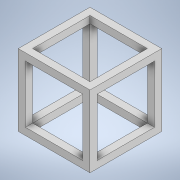
# Autodesk Inventor part: Hollow_Cube
Saved by Autodesk Inventor 2020 (Build 240168000, 168)
## iProperties
Created: 2021-12-24
Part Number: Hollow_Cube
Material: Generic
Document SubType Name: Modeling
Designer: Umur Batuhan Özmen
Density: 1 g/cm^3
Appearance: Default
Author: Umur Batuhan Özmen
Autodesk Inventor part; units mm, degrees
ref_plane "YZ Plane" through (0, 0, 0) normal (1, 0, 0) x (0, 1, 0)
ref_plane "XZ Plane" through (0, 0, 0) normal (0, 1, 0) x (-1, 0, 0)
ref_plane "XY Plane" through (0, 0, 0) normal (0, 0, 1) x (1, 0, 0)
sketch "Sketch1" plane through (0, 0, 0) normal (0, 1, 0) x (-1, 0, 0)
  line L0 (50, 50) -> (-50, 50)
  line L1 (-50, 50) -> (-50, -50)
  line L2 (-50, -50) -> (50, -50)
  line L3 (50, -50) -> (50, 50)
  line L4 (50, 50) -> (-50, -50) construction
  line L5 (-50, 50) -> (50, -50) construction
  line L6 (40, 40) -> (-40, 40)
  line L7 (-40, 40) -> (-40, -40)
  line L8 (-40, -40) -> (40, -40)
  line L9 (40, -40) -> (40, 40)
  line L10 (40, 40) -> (-40, -40) construction
  line L11 (-40, 40) -> (40, -40) construction
  point P0 (0, 0)
  dimension "d0" = 100
  dimension "d1" = 100
  dimension "d2" = 80
  dimension "d3" = 80
  constraints: 24 end point, 4 midpoint, 4 parallel, 2 horizontal, 2 perpendicular
  measures "d0" distance of L2.end L1.end
  measures "d1" distance of L1.end L0.end
  measures "d2" distance of L8.end L7.end
  measures "d3" distance of L7.end L6.end
extrude "Extrusion1" add sketch "Sketch1" along normal blind 10
sketch "Sketch2" plane through (0, 10, 0) normal (0, 1, 0) x (1, 0, 0)
  line L0 (40, -40) -> (50, -40)
  line L1 (50, -40) -> (50, -50)
  line L2 (50, -50) -> (40, -50)
  line L3 (40, -50) -> (40, -40)
  line L4 (40, 40) -> (40, -40) projected
  line L5 (50, 50) -> (-50, 50) projected
  line L6 (40, 40) -> (50, 40)
  line L7 (50, 40) -> (50, 50)
  line L8 (50, 50) -> (40, 50)
  line L9 (40, 50) -> (40, 40)
  line L10 (-40, -40) -> (-40, 40) projected
  line L11 (-50, 50) -> (-50, -50) projected
  line L12 (-40, 40) -> (-50, 40)
  line L13 (-50, 40) -> (-50, 50)
  line L14 (-50, 50) -> (-40, 50)
  line L15 (-40, 50) -> (-40, 40)
  line L16 (40, -40) -> (-40, -40) projected
  line L17 (-40, -40) -> (-50, -40)
  line L18 (-50, -40) -> (-50, -50)
  line L19 (-50, -50) -> (-40, -50)
  line L20 (-40, -50) -> (-40, -40)
  point P0 (0, 0)
  constraints: 32 end point, 8 parallel, 4 horizontal, 4 perpendicular, 2 point on line
extrude "Extrusion2" add sketch "Sketch2" along normal blind 80 contours L0 L1 L2 L3 | L9 L5 L7 L6 | L20 L19 L11 L17 | L12 L11 L5 L15
sketch "Sketch3" plane through (0, 90, 0) normal (0, 1, 0) x (1, 0, 0)
  line L0 (-50, -50) -> (50, -50)
  line L1 (50, -50) -> (50, 50)
  line L2 (50, 50) -> (-50, 50)
  line L3 (-50, 50) -> (-50, -50)
  line L4 (-50, -50) -> (50, 50) construction
  line L5 (50, -50) -> (-50, 50) construction
  line L6 (-40, -40) -> (40, -40)
  line L7 (40, -40) -> (40, 40)
  line L8 (40, 40) -> (-40, 40)
  line L9 (-40, 40) -> (-40, -40)
  line L10 (-40, -40) -> (40, 40) construction
  line L11 (40, -40) -> (-40, 40) construction
  point P0 (0, 0)
  dimension "d8" = 100
  dimension "d9" = 100
  dimension "d10" = 80
  dimension "d11" = 80
  constraints: 24 end point, 4 midpoint, 4 parallel, 2 horizontal, 2 perpendicular
  measures "d8" distance of L2.end L1.end
  measures "d9" distance of L1.end L0.end
  measures "d10" distance of L8.end L7.end
  measures "d11" distance of L7.end L6.end
extrude "Extrusion3" add sketch "Sketch3" along normal blind 10
body "Solid1"
